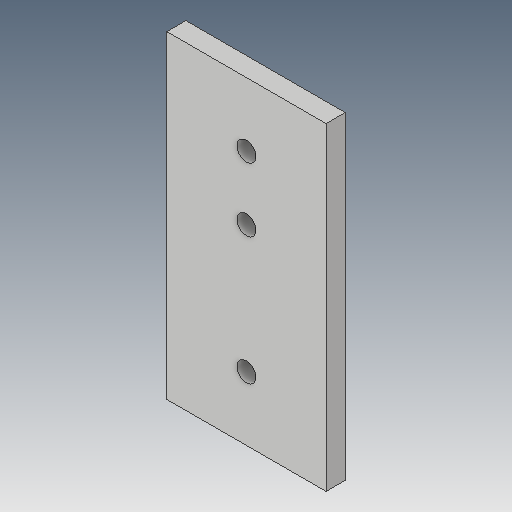
# Autodesk Inventor part: plat sim
Saved by Autodesk Inventor 2018 (Build 220112000, 112)
## iProperties
Created: 2019-12-19
Part Number: plat sim
Material: Generic
Document SubType Name: Modeling
Designer: Ibnu
Density: 1 g/cm^3
Appearance: Default
Mass: 3.68638 g
Surface Area: 29.9241 cm^2
Volume: 3.68638 cm^3
Author: Ibnu
Autodesk Inventor part; units mm, degrees
ref_plane "YZ Plane" through (0, 0, 0) normal (1, 0, 0) x (0, 1, 0)
ref_plane "XZ Plane" through (0, 0, 0) normal (0, 1, 0) x (-1, 0, 0)
ref_plane "XY Plane" through (0, 0, 0) normal (0, 0, 1) x (1, 0, 0)
sketch "Sketch1" plane through (0, 0, 0) normal (0, 0, 1) x (1, 0, 0)
  line L0 (0, 0) -> (25, 0)
  line L1 (25, 0) -> (25, -50)
  line L2 (0, -50) -> (0, 0)
  circle A0 centre (12.5, -40) radius 1.5
  circle A1 centre (12.5, -20) radius 1.5
  circle A2 centre (12.5, -10) radius 1.5
  line L3 (12.5, -50) -> (0, -50)
  line L4 (12.5, -50) -> (25, -50)
  dimension "d6" = 3
  dimension "d7" = 3
  constraints: 10 end point, 3 centre point, 2 horizontal, 1 parallel, 1 perpendicular, 1 point on line
  measures "d6" diameter of A1
  measures "d7" diameter of A2
extrude "Extrusion1" add sketch "Sketch1" along normal blind 3
body "Solid1"
